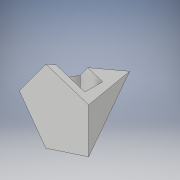
# Autodesk Inventor part: Шар
Saved by Autodesk Inventor 2019.3 (Build 233278000, 278)
## iProperties
Created: 2020-04-03
Part Number: Шар
Material: Типовые
Document SubType Name: Modeling
Designer: Admin
Density: 1 g/cm^3
Appearance: По умолчанию
Author: Admin
Autodesk Inventor part; units mm, degrees
ref_plane "YZ Plane" through (0, 0, 0) normal (1, 0, 0) x (0, 1, 0)
ref_plane "XZ Plane" through (0, 0, 0) normal (0, 1, 0) x (-1, 0, 0)
sketch "Эскиз1" plane through (0, 0, 0) normal (0, 0, 1) x (1, 0, 0)
  line L0 (-42.5, 0) -> (-13.1332, 40.4199)
  line L1 (-13.1332, 40.4199) -> (34.3832, 24.9809)
  line L2 (34.3832, 24.9809) -> (34.3832, -24.9809)
  line L3 (34.3832, -24.9809) -> (-13.1332, -40.4199)
  line L4 (-13.1332, -40.4199) -> (-42.5, 0)
  point P0 (0, 0)
  point P1 (0, 0)
  constraints: 10 end point, 1 coincident, 1 horizontal alignment, 11 other
sketch "Эскиз2" plane through (0, 0, 0) normal (0, 1, 0) x (-1, 0, 0)
  line L0 (30, -10) -> (-20, -10)
  line L1 (-20, -10) -> (-10, -40)
  line L2 (-10, -40) -> (15, -40)
  line L3 (15, -40) -> (30, -10)
  line L4 (13.1332, 0) -> (-34.3832, 0) projected
  line L5 (42.5, 0) -> (13.1332, 0) projected
  point P0 (0, 0)
  dimension "d1" = 10
  dimension "d2" = 30
  dimension "d3" = 10
  dimension "d4" = 20
  dimension "d5" = 50
  dimension "d6" = 25
  constraints: 8 end point, 2 horizontal
  measures "d1" horizontal distance of point (0, 0) L1.end
  measures "d2" distance between parallel lines of L2 L0
  measures "d3" distance between parallel lines of L4 L0
  measures "d4" horizontal distance of point (0, 0) L0.end
  measures "d5" distance of L0.start L0.end
  measures "d6" distance of L1.end L2.end
ref_plane "РабПлоскость1" through (0, 0, -80) normal (0, 0, 1) x (1, 0, 0)
sketch "Эскиз3" plane through (0, 0, -80) normal (0, 0, 1) x (1, 0, 0)
  point P0 (0, 0)
  point P1 (0, 0)
  point P2 (0, 0)
  constraints: 1 coincident
loft "Лофт1" add profiles "Эскиз1" section 2 point at (0, 0, -80)
extrude "Выдавливание1" cut sketch "Эскиз2" along normal through all both and the other way through all
